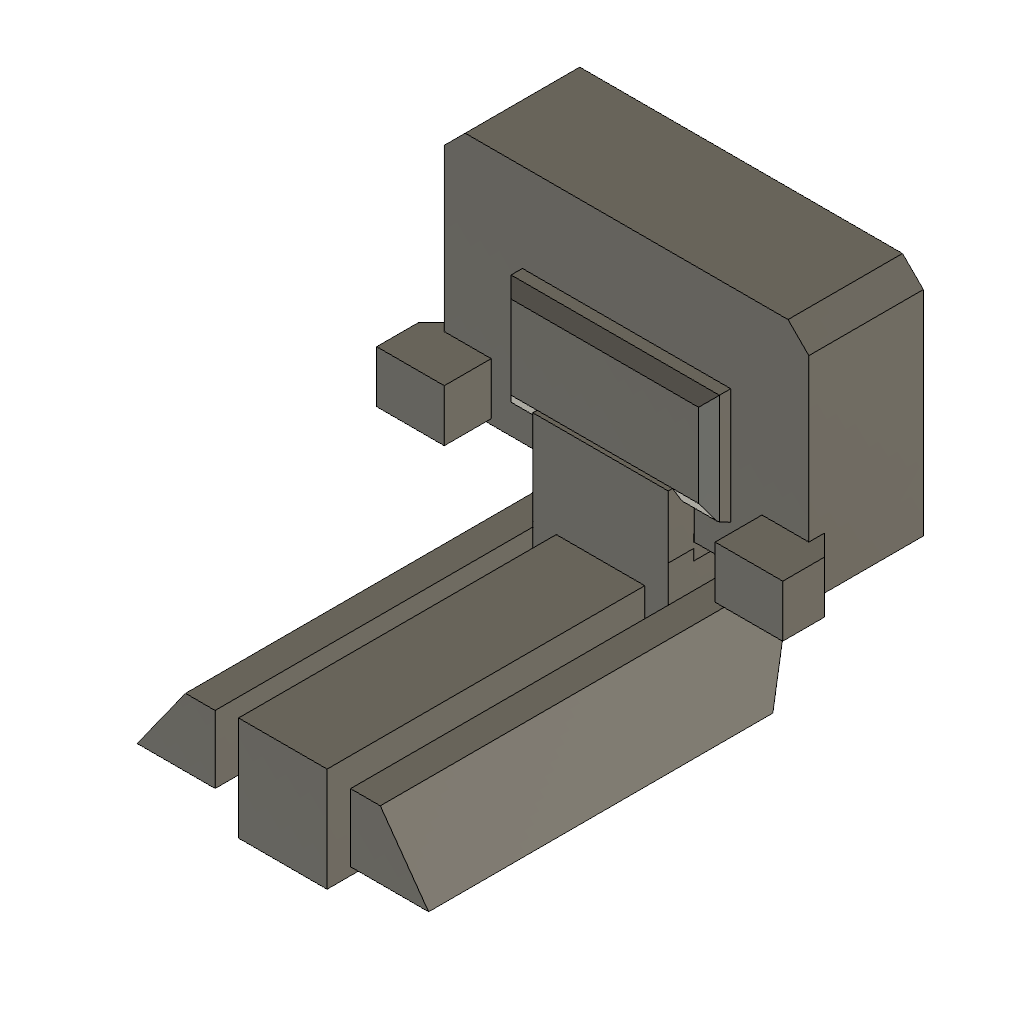
R9_G20_button_1_RIGHT_TF (Autodesk Fusion 360 design; units mm, degrees)
part number: 2026-10-05-03-56-05-775
Autodesk Fusion 360 part; units mm, degrees
ref_plane "工作平面1" through (0, -32.4, 0) normal (0, 1, 0) x (0, 0, 1)
sketch "草图1" plane through (0, -32.4, 0) normal (0, 1, 0) x (1, 0, 0)
  line L0 (-9.1958, 7.3, 64.8) -> (-3.7958, 7.3, 64.8)
  line L1 (-3.7958, 7.3, 64.8) -> (-3.4958, 7, 64.8)
  line L2 (-3.4958, 7, 64.8) -> (-3.4958, 3.5, 64.8)
  line L3 (-3.4958, 3.5, 64.8) -> (-3.7958, 3.2, 64.8)
  line L4 (-3.7958, 3.2, 64.8) -> (-9.1958, 3.2, 64.8)
  line L5 (-9.1958, 3.2, 64.8) -> (-9.4958, 3.5, 64.8)
  line L6 (-9.4958, 3.5, 64.8) -> (-9.4958, 7, 64.8)
  line L7 (-9.4958, 7, 64.8) -> (-9.1958, 7.3, 64.8)
extrude "R6 rounded corner cap recessed 0.10mm" add sketch "草图1" along normal blind 2.2 contours L0 L1 L2 L3 L4 L5 L6 L7 in plane through (0, 32.4, 0) normal (0, 1, 0)
ref_plane "工作平面2" through (0, -31.9, 0) normal (0, 1, 0) x (0, 0, 1)
sketch "草图2" plane through (0, -31.9, 0) normal (0, 1, 0) x (1, 0, 0)
  line L0 (-9.2958, 9.5, 63.8) -> (-3.6958, 9.5, 63.8)
  line L1 (-3.6958, 9.5, 63.8) -> (-4.6958, 8.1, 63.8)
  line L2 (-4.6958, 8.1, 63.8) -> (-5.1958, 8.1, 63.8)
  line L3 (-5.1958, 8.1, 63.8) -> (-5.1958, 7.25, 63.8)
  line L4 (-5.1958, 7.25, 63.8) -> (-7.7958, 7.25, 63.8)
  line L5 (-7.7958, 7.25, 63.8) -> (-7.7958, 8.1, 63.8)
  line L6 (-7.7958, 8.1, 63.8) -> (-8.2958, 8.1, 63.8)
  line L7 (-8.2958, 8.1, 63.8) -> (-9.2958, 9.5, 63.8)
extrude "R6 track compatible dovetail neck" add sketch "草图2" along normal blind 2.7 contours L0 L1 L2 L3 L4 L5 L6 L7 in plane through (0, 31.9, 0) normal (0, 1, 0)
ref_plane "工作平面3" through (-9.5958, 0, 0) normal (1, 0, 0) x (0, 1, 0)
sketch "草图3" plane through (-9.5958, 0, 0) normal (1, 0, 0) x (0, 0, -1)
  line L0 (9.51, 32.4) -> (9.51, 34.61)
  line L1 (9.51, 34.61) -> (7.29, 34.61)
  line L2 (7.29, 34.61) -> (9.51, 32.4)
extrude "R6 45deg lower neck printing relief" cut sketch "草图3" along normal blind 6.2
ref_plane "工作平面4" through (0, -25.8, 0) normal (0, 1, 0) x (0, 0, 1)
sketch "草图4" plane through (0, -25.8, 0) normal (0, 1, 0) x (1, 0, 0)
  line L0 (-7.7958, 9.5, 51.6) -> (-9.2958, 9.5, 51.6)
  line L1 (-9.2958, 9.5, 51.6) -> (-8.2958, 8.1, 51.6)
  line L2 (-8.2958, 8.1, 51.6) -> (-7.7958, 8.1, 51.6)
  line L3 (-7.7958, 8.1, 51.6) -> (-7.7958, 9.5, 51.6)
extrude "R6 6.3mm guide runner -1" add sketch "草图4" along normal blind 6.3 contours L0 L1 L2 L3 in plane through (0, 25.8, 0) normal (0, 1, 0)
ref_plane "工作平面5" through (0, 0, -7.3) normal (0, 0, 1) x (1, 0, 0)
sketch "草图5" plane through (0, 0, -7.3) normal (0, 0, 1) x (1, 0, 0)
  line L0 (-9.0958, 31.5) -> (-10.3958, 31.5)
  line L1 (-10.3958, 31.5) -> (-10.3958, 32.3)
  line L2 (-10.3958, 32.3) -> (-9.4958, 33.2)
  line L3 (-9.4958, 33.2) -> (-9.0958, 33.2)
  line L4 (-9.0958, 33.2) -> (-9.0958, 31.5)
extrude "R6 shoulder above rail roof -1" add sketch "草图5" along normal blind 1
ref_plane "工作平面6" through (0, -25.8, 0) normal (0, 1, 0) x (0, 0, 1)
sketch "草图6" plane through (0, -25.8, 0) normal (0, 1, 0) x (1, 0, 0)
  line L0 (-5.1958, 9.5, 51.6) -> (-3.6958, 9.5, 51.6)
  line L1 (-3.6958, 9.5, 51.6) -> (-4.6958, 8.1, 51.6)
  line L2 (-4.6958, 8.1, 51.6) -> (-5.1958, 8.1, 51.6)
  line L3 (-5.1958, 8.1, 51.6) -> (-5.1958, 9.5, 51.6)
extrude "R6 6.3mm guide runner 1" add sketch "草图6" along normal blind 6.3 contours L0 L1 L2 L3 in plane through (0, 25.8, 0) normal (0, 1, 0)
ref_plane "工作平面7" through (0, 0, -7.3) normal (0, 0, 1) x (1, 0, 0)
sketch "草图7" plane through (0, 0, -7.3) normal (0, 0, 1) x (1, 0, 0)
  line L0 (-3.8958, 31.5) -> (-2.5958, 31.5)
  line L1 (-2.5958, 31.5) -> (-2.5958, 32.3)
  line L2 (-2.5958, 32.3) -> (-3.4958, 33.2)
  line L3 (-3.4958, 33.2) -> (-3.8958, 33.2)
  line L4 (-3.8958, 33.2) -> (-3.8958, 31.5)
extrude "R6 shoulder above rail roof 1" add sketch "草图7" along normal blind 1
ref_plane "工作平面8" through (0, 0, -9.1) normal (0, 0, 1) x (1, 0, 0)
sketch "草图8" plane through (0, 0, -9.1) normal (0, 0, 1) x (1, 0, 0)
  line L0 (-7.3458, 25.8) -> (-5.6458, 25.8)
  line L1 (-5.6458, 25.8) -> (-5.6458, 32.05)
  line L2 (-5.6458, 32.05) -> (-7.3458, 32.05)
  line L3 (-7.3458, 32.05) -> (-7.3458, 25.8)
extrude "R6 1mm assembly latch leaf" add sketch "草图8" along normal blind 1
ref_plane "工作平面9" through (-7.3458, 0, 0) normal (1, 0, 0) x (0, 1, 0)
sketch "草图9" plane through (-7.3458, 0, 0) normal (1, 0, 0) x (0, 0, -1)
  line L0 (10.1, 25.8) -> (10.1, 26.4)
  line L1 (10.1, 26.4) -> (9.1, 27.4)
  line L2 (9.1, 27.4) -> (9.1, 25.8)
  line L3 (9.1, 25.8) -> (10.1, 25.8)
extrude "R6 45deg latch ramp" add sketch "草图9" along normal blind 1.7
ref_plane "工作平面10" through (-7.3958, 0, 0) normal (1, 0, 0) x (0, 1, 0)
sketch "草图10" plane through (-7.3958, 0, 0) normal (1, 0, 0) x (0, 0, -1)
  line L0 (7.3, 33.5) -> (4.9, 33.5)
  line L1 (4.9, 33.5) -> (4.9, 31.9826)
  line L2 (4.9, 31.9826) -> (6.1, 31.9826)
  line L3 (6.1, 31.9826) -> (7.3, 33.5)
extrude "R6 centered switch contact" add sketch "草图10" along normal blind 1.8
ref_plane "工作平面11" through (0, 0, -7.5) normal (0, 0, 1) x (1, 0, 0)
sketch "草图11" plane through (0, 0, -7.5) normal (0, 0, 1) x (1, 0, 0)
  line L0 (-7.8058, 31.89) -> (-5.1858, 31.89)
  line L1 (-5.1858, 31.89) -> (-5.1858, 32.39)
  line L2 (-5.1858, 32.39) -> (-7.8058, 32.39)
  line L3 (-7.8058, 32.39) -> (-7.8058, 31.89)
extrude "R6 rear neck switch body clearance 1" cut sketch "草图11" along normal blind 0.26
ref_plane "工作平面12" through (0, 0, -8.2) normal (0, 0, 1) x (1, 0, 0)
sketch "草图12" plane through (0, 0, -8.2) normal (0, 0, 1) x (1, 0, 0)
  line L0 (-9.5058, 25.79) -> (-7.7958, 25.79)
  line L1 (-7.7958, 25.79) -> (-7.7958, 34.39)
  line L2 (-7.7958, 34.39) -> (-9.5058, 34.39)
  line L3 (-9.5058, 34.39) -> (-9.5058, 25.79)
extrude "R6 guide vertical 0.35mm clearance 1 -1" cut sketch "草图12" along normal blind 0.11
ref_plane "工作平面13" through (0, 0, -8.2) normal (0, 0, 1) x (1, 0, 0)
sketch "草图13" plane through (0, 0, -8.2) normal (0, 0, 1) x (1, 0, 0)
  line L0 (-5.1958, 25.79) -> (-3.4858, 25.79)
  line L1 (-3.4858, 25.79) -> (-3.4858, 34.39)
  line L2 (-3.4858, 34.39) -> (-5.1958, 34.39)
  line L3 (-5.1958, 34.39) -> (-5.1958, 25.79)
extrude "R6 guide vertical 0.35mm clearance 1 1" cut sketch "草图13" along normal blind 0.11
ref_plane "工作平面14" through (0, -32.4, 0) normal (0, 1, 0) x (0, 0, 1)
sketch "草图14" plane through (0, -32.4, 0) normal (0, 1, 0) x (1, 0, 0)
  line L0 (-9.4458, 7.6, 64.8) -> (-3.5458, 7.6, 64.8)
  line L1 (-3.5458, 7.6, 64.8) -> (-3.1958, 7.25, 64.8)
  line L2 (-3.1958, 7.25, 64.8) -> (-3.1958, 3.25, 64.8)
  line L3 (-3.1958, 3.25, 64.8) -> (-3.5458, 2.9, 64.8)
  line L4 (-3.5458, 2.9, 64.8) -> (-9.4458, 2.9, 64.8)
  line L5 (-9.4458, 2.9, 64.8) -> (-9.7958, 3.25, 64.8)
  line L6 (-9.7958, 3.25, 64.8) -> (-9.7958, 7.25, 64.8)
  line L7 (-9.7958, 7.25, 64.8) -> (-9.4458, 7.6, 64.8)
extrude "R7A cap 6.60 x 4.70 mm - unchanged 0.10 recess" add sketch "草图14" along normal blind 2.2 contours L0 L1 L2 L3 L4 L5 L6 L7 in plane through (0, 32.4, 0) normal (0, 1, 0)
ref_plane "工作平面15" through (0, -26.1, 0) normal (0, 1, 0) x (0, 0, 1)
sketch "草图15" plane through (0, -26.1, 0) normal (0, 1, 0) x (1, 0, 0)
  line L0 (-7.7958, 9.5, 52.2) -> (-9.3958, 9.5, 52.2)
  line L1 (-9.3958, 9.5, 52.2) -> (-8.3958, 8.1, 52.2)
  line L2 (-8.3958, 8.1, 52.2) -> (-7.7958, 8.1, 52.2)
  line L3 (-7.7958, 8.1, 52.2) -> (-7.7958, 9.5, 52.2)
ref_plane "工作平面16" through (0, -26.1, 0) normal (0, 1, 0) x (0, 0, 1)
sketch "草图16" plane through (0, -26.1, 0) normal (0, 1, 0) x (1, 0, 0)
  line L0 (-5.1958, 9.5, 52.2) -> (-3.5958, 9.5, 52.2)
  line L1 (-3.5958, 9.5, 52.2) -> (-4.5958, 8.1, 52.2)
  line L2 (-4.5958, 8.1, 52.2) -> (-5.1958, 8.1, 52.2)
  line L3 (-5.1958, 8.1, 52.2) -> (-5.1958, 9.5, 52.2)
ref_plane "工作平面17" through (0, -32.4, 0) normal (0, 1, 0) x (0, 0, 1)
sketch "草图17" plane through (0, -32.4, 0) normal (0, 1, 0) x (1, 0, 0)
  line L0 (-9.4959, 7.6, 64.8) -> (-3.4959, 7.6, 64.8)
  line L1 (-3.4959, 7.6, 64.8) -> (-3.0959, 7.2, 64.8)
  line L2 (-3.0959, 7.2, 64.8) -> (-3.0959, 3.3, 64.8)
  line L3 (-3.0959, 3.3, 64.8) -> (-3.4959, 2.9, 64.8)
  line L4 (-3.4959, 2.9, 64.8) -> (-9.4959, 2.9, 64.8)
  line L5 (-9.4959, 2.9, 64.8) -> (-9.8959, 3.3, 64.8)
  line L6 (-9.8959, 3.3, 64.8) -> (-9.8959, 7.2, 64.8)
  line L7 (-9.8959, 7.2, 64.8) -> (-9.4959, 7.6, 64.8)
extrude "R8 visible cap 6.8x4.7 separate from 0.35 guide" add sketch "草图17" along normal blind 2.2 contours L0 L1 L2 L3 L4 L5 L6 L7 in plane through (0, 32.4, 0) normal (0, 1, 0)
ref_plane "工作平面18" through (0, 0, -7.4) normal (0, 0, 1) x (1, 0, 0)
sketch "草图18" plane through (0, 0, -7.4) normal (0, 0, 1) x (1, 0, 0)
  line L0 (-7.5059, 30) -> (-5.4859, 30)
  line L1 (-5.4859, 30) -> (-5.4859, 32.4001)
  line L2 (-5.4859, 32.4001) -> (-7.5059, 32.4001)
  line L3 (-7.5059, 32.4001) -> (-7.5059, 30)
extrude "R8 remove old narrow contact nose" cut sketch "草图18" along normal blind 2.6
ref_plane "工作平面19" through (-8.4959, 0, 0) normal (1, 0, 0) x (0, 1, 0)
sketch "草图19" plane through (-8.4959, 0, 0) normal (1, 0, 0) x (0, 0, -1)
  line L0 (7.3, 33.5) -> (4.5, 33.5)
  line L1 (4.5, 33.5) -> (4.5, 31.9827)
  line L2 (4.5, 31.9827) -> (6.5, 31.9827)
  line L3 (6.5, 31.9827) -> (7.3, 33.5)
extrude "R8 broad centered contact 4x2 G20" add sketch "草图19" along normal blind 4
chamfer "倒角1" distance 0.2 angle 45 4 edges at (-6.4959, 31.9827, -6.5) (-8.4959, 31.9827, -5.5) (-4.4959, 31.9827, -5.5) (-6.4959, 31.9827, -4.5) tangent chain off
ref_plane "工作平面20" through (0, -32.4, 0) normal (0, 1, 0) x (0, 0, 1)
sketch "草图20" plane through (0, -32.4, 0) normal (0, 1, 0) x (1, 0, 0)
  line L0 (-9.4959, 7.7, 64.8) -> (-3.4959, 7.7, 64.8)
  line L1 (-3.4959, 7.7, 64.8) -> (-3.0959, 7.3, 64.8)
  line L2 (-3.0959, 7.3, 64.8) -> (-3.0959, 3.2, 64.8)
  line L3 (-3.0959, 3.2, 64.8) -> (-3.4959, 2.8, 64.8)
  line L4 (-3.4959, 2.8, 64.8) -> (-9.4959, 2.8, 64.8)
  line L5 (-9.4959, 2.8, 64.8) -> (-9.8959, 3.2, 64.8)
  line L6 (-9.8959, 3.2, 64.8) -> (-9.8959, 7.3, 64.8)
  line L7 (-9.8959, 7.3, 64.8) -> (-9.4959, 7.7, 64.8)
extrude "R8 FINAL cap 6.8x4.9 - four straight edge gaps 0.20" add sketch "草图20" along normal blind 2.2 contours L0 L1 L2 L3 L4 L5 L6 L7 in plane through (0, 32.4, 0) normal (0, 1, 0)
ref_plane "工作平面21" through (-9.9959, 0, 0) normal (1, 0, 0) x (0, 1, 0)
sketch "草图21" plane through (-9.9959, 0, 0) normal (1, 0, 0) x (0, 0, -1)
  line L0 (7.71, 32.39) -> (7.71, 34)
  line L1 (7.71, 34) -> (7.4, 33.69)
  line L2 (7.4, 33.69) -> (7.4, 32.39)
  line L3 (7.4, 32.39) -> (7.71, 32.39)
extrude "R8 rear underside assembly relief - full visible cap retained" cut sketch "草图21" along normal blind 7
ref_plane "工作平面22" through (0, -32.4, 0) normal (0, 1, 0) x (0, 0, 1)
sketch "草图22" plane through (0, -32.4, 0) normal (0, 1, 0) x (1, 0, 0)
  line L0 (-9.5959, 7.7, 64.8) -> (-3.3959, 7.7, 64.8)
  line L1 (-3.3959, 7.7, 64.8) -> (-2.9959, 7.3, 64.8)
  line L2 (-2.9959, 7.3, 64.8) -> (-2.9959, 3.2, 64.8)
  line L3 (-2.9959, 3.2, 64.8) -> (-3.3959, 2.8, 64.8)
  line L4 (-3.3959, 2.8, 64.8) -> (-9.5959, 2.8, 64.8)
  line L5 (-9.5959, 2.8, 64.8) -> (-9.9959, 3.2, 64.8)
  line L6 (-9.9959, 3.2, 64.8) -> (-9.9959, 7.3, 64.8)
  line L7 (-9.9959, 7.3, 64.8) -> (-9.5959, 7.7, 64.8)
extrude "R9 visible cap WIDTH 7.0 HEIGHT unchanged 4.9" add sketch "草图22" along normal blind 2.2 contours L0 L1 L2 L3 L4 L5 L6 L7 in plane through (0, 32.4, 0) normal (0, 1, 0)
ref_plane "工作平面23" through (-10.0959, 0, 0) normal (1, 0, 0) x (0, 1, 0)
sketch "草图23" plane through (-10.0959, 0, 0) normal (1, 0, 0) x (0, 0, -1)
  line L0 (7.71, 32.39) -> (7.71, 34)
  line L1 (7.71, 34) -> (7.4, 33.69)
  line L2 (7.4, 33.69) -> (7.4, 32.39)
  line L3 (7.4, 32.39) -> (7.71, 32.39)
extrude "R9 preserve hidden outer assembly relief" cut sketch "草图23" along normal blind 7.2
ref_plane "工作平面24" through (0, 0, -8.1) normal (0, 0, 1) x (1, 0, 0)
sketch "草图24" plane through (0, 0, -8.1) normal (0, 0, 1) x (1, 0, 0)
  line L0 (-7.7959, 31.9) -> (-5.1959, 31.9)
  line L1 (-5.1959, 31.9) -> (-5.1959, 33.5)
  line L2 (-5.1959, 33.5) -> (-7.7959, 33.5)
  line L3 (-7.7959, 33.5) -> (-7.7959, 31.9)
extrude "R9 central connection web 2.6 wide x 1.8 high x 1.6 long" add sketch "草图24" along normal blind 1.8
